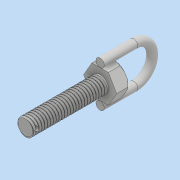
# Autodesk Inventor part: Bolt
Saved by Autodesk Inventor 2018 (Build 220112000, 112)
## iProperties
Created: 2020-08-11
Part Number: Bolt
Material: Generic
Document SubType Name: Modeling
Designer: ASUS
Density: 1 g/cm^3
Appearance: Default
Author: ASUS
Autodesk Inventor part; units mm, degrees
ref_plane "YZ Plane" through (0, 0, 0) normal (1, 0, 0) x (0, 1, 0)
ref_plane "XZ Plane" through (0, 0, 0) normal (0, 1, 0) x (-1, 0, 0)
ref_plane "XY Plane" through (0, 0, 0) normal (0, 0, 1) x (1, 0, 0)
sketch "Sketch3" plane through (0, 0, 0) normal (0, 1, 0) x (-1, 0, 0)
  line L0 (-4.9048, -8.5016) -> (-9.815, -0.0031)
  line L1 (-9.815, -0.0031) -> (-4.9102, 8.4984)
  line L2 (-4.9102, 8.4984) -> (4.9048, 8.5016)
  line L3 (4.9048, 8.5016) -> (9.815, 0.0031)
  line L4 (9.815, 0.0031) -> (4.9102, -8.4984)
  line L5 (4.9102, -8.4984) -> (-4.9048, -8.5016)
  point P0 (0, 0)
  point P1 (0, 0)
  dimension "d1" = 17
  constraints: 12 end point, 1 coincident, 13 other
  measures "d1" distance between parallel lines of L2 L5
extrude "Extrusion1" add sketch "Sketch3" along normal blind 8
sketch "Sketch4" plane through (0, 8, 0) normal (0, 1, 0) x (1, 0, 0)
  circle A0 centre (0, 0) radius 8.6061
  constraints: 1 centre point, 1 coincident
extrude "Extrusion2" cut sketch "Sketch4" against normal through all draft 45 keep common part
sketch "Sketch5" plane through (0, 0, 0) normal (0, -1, 0) x (1, 0, 0)
  circle A0 centre (0, 0) radius 5
  dimension "d6" = 10
  constraints: 1 centre point, 1 coincident
  measures "d6" diameter of A0
extrude "Extrusion3" add sketch "Sketch5" along normal blind 45
sketch "Sketch6" plane through (0, 0, 0) normal (1, 0, 0) x (0, 1, 0)
  line L0 (-47, 5) -> (-48.5, 5)
  line L1 (-45, 5) -> (-45, -5) projected
  line L2 (-48.5, 5) -> (-47.9232, 4.001)
  line L3 (-48.5, 5) -> (-46.3699, 5) construction
  line L4 (-47, 5) -> (-47.5768, 4.001)
  line L5 (-47, 5) -> (-44, 5) construction
  arc A0 (-47.9232, 4.001) -> (-47.5768, 4.001) centre (-47.75, 4.101) ccw
  point P0 (0, 0)
  dimension "d10" = 1.5
  dimension "d11" = 2
  dimension "d12" = 60
  dimension "d13" = 120
  dimension "d14" = 0.2
  constraints: 10 end point, 3 horizontal, 2 point on circle, 2 tangent, 1 centre point
  measures "d10" distance of L0.start L0.end
  measures "d11" distance from line of L1 L0.start
  measures "d12" angle of L2 L3
  measures "d13" angle of L4 L5
  measures "d14" radius of A0
coil "Coil2" sketch "Sketch6" operation cut axis through (0, -10, 0) along (0, 1, 0) pitch 1.7 turns 27.647059 hand right
sketch "Sketch18" plane through (0, 0, 0) normal (1, 0, 0) x (0, 1, 0)
  line L0 (0, 11) -> (20, 11)
  line L1 (0, -11) -> (20, -11) construction
  line L2 (0, -0.0031) -> (6.7911, -0.0031) projected
  arc A0 (20, -11) -> (20, 11) centre (20, 0) ccw
  line L3 (20, -11) -> (0, -11)
  line L4 (0, -0.0031) -> (0, 8.4984) projected
  point P0 (0, 0)
  dimension "d92" = 20
  dimension "d95" = 11.0031
  dimension "d97" = 11
  dimension "d101" = 20
  dimension "d102" = 0
  constraints: 6 end point, 2 horizontal, 2 point on circle, 1 centre point, 1 collinear
  measures "d92" distance of L0.start L0.end
  measures "d95" distance between parallel lines of L2 L0
  measures "d97" radius of A0
  measures "d101" distance of L1.start L1.end
  measures "d102" distance from line of L4 L0.start
sketch "Sketch19" plane through (0, 0, 0) normal (0, -1, 0) x (1, 0, 0)
  circle A0 centre (0, 11) radius 2.5
  point P0 (0, 0)
  dimension "d98" = 5
  constraints: 1 centre point
  measures "d98" diameter of A0
sweep "Sweep1" add profiles "Sketch19" path "Sketch18" path curves L0 A0 L3
sketch "Sketch20" plane through (0, 0, 0) normal (1, 0, 0) x (0, 1, 0)
  circle A0 centre (-42, 0) radius 1.5
  point P0 (0, 0)
  dimension "d103" = 3
  constraints: 1 centre point
  measures "d103" diameter of A0
extrude "Extrusion11" cut sketch "Sketch20" along normal mid plane 28
body "Solid1"
